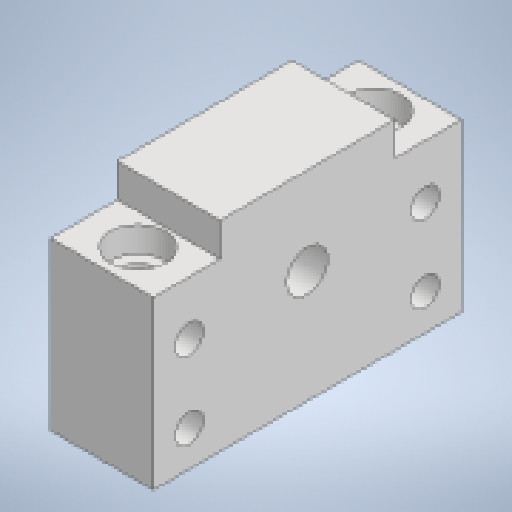
# Autodesk Inventor part: BF10
Saved by Autodesk Inventor 2023 (Build 270158000, 158)
## iProperties
Created: 2022-04-29
Part Number: BF10
Material: Generic
Document SubType Name: Modeling
Designer: plebbb
Density: 1 g/cm^3
Appearance: Default
Author: plebbb
Autodesk Inventor part; units mm, degrees
ref_plane "YZ Plane" through (0, 0, 0) normal (1, 0, 0) x (0, 1, 0)
ref_plane "XZ Plane" through (0, 0, 0) normal (0, 1, 0) x (-1, 0, 0)
ref_plane "XY Plane" through (0, 0, 0) normal (0, 0, 1) x (1, 0, 0)
sketch "Sketch1" plane through (0, 0, 0) normal (1, 0, 0) x (0, 1, 0)
  line L0 (0, 0) -> (32.5, 0)
  line L1 (32.5, 0) -> (32.5, -13)
  line L2 (32.5, -13) -> (39, -13)
  line L3 (39, -13) -> (39, -47)
  line L4 (39, -47) -> (32.5, -47)
  line L5 (32.5, -47) -> (32.5, -60)
  line L6 (32.5, -60) -> (0, -60)
  line L7 (0, -60) -> (0, 0)
  circle A0 centre (22, -53) radius 2.75
  circle A1 centre (7, -7) radius 2.75
  circle A2 centre (7, -53) radius 2.75
  circle A3 centre (22, -7) radius 2.75
  line L8 (22, -7) -> (7, -7) construction
  line L9 (7, -7) -> (7, -53) construction
  line L10 (7, -53) -> (22, -53) construction
  line L11 (22, -53) -> (22, -7) construction
  line L12 (7, -30) -> (0, -30) construction
  circle A4 centre (22, -30) radius 4
  dimension "d0" = 34
  dimension "d1" = 60
  dimension "d2" = 39
  dimension "d3" = 32.5
  dimension "d4" = 5.5
  dimension "d6" = 22
  dimension "d7" = 15
  dimension "d8" = 46
  dimension "d9" = 8
  constraints: 26 end point, 8 perpendicular, 5 centre point, 4 coincident, 4 midpoint, 3 equal radius, 2 horizontal, 2 parallel, 2 point on line, 1 collinear
  measures "d0" distance of L2.end L3.end
  measures "d1" distance between parallel lines of L6 L0
  measures "d2" distance between parallel lines of L7 L3
  measures "d3" distance from line of L0.start L1
  measures "d4" diameter of A3
  measures "d6" horizontal distance of L6.end A0.centre
  measures "d7" distance of L9.end L10.end
  measures "d8" distance of L8.end L9.end
  measures "d9" diameter of A4
extrude "Extrusion1" add sketch "Sketch1" along normal blind 20
sketch "Sketch2" plane through (0, 32.5, 0) normal (0, 1, 0) x (1, 0, 0)
  circle A0 centre (10, 7) radius 5.4
  circle A1 centre (10, 53) radius 5.4
  point P0 (0, 0)
  dimension "d12" = 10.8
  dimension "d13" = 10.8
  dimension "d14" = 46
  dimension "d15" = 7
  dimension "d16" = 10
  constraints: 2 centre point, 1 vertical alignment
  measures "d12" diameter of A0
  measures "d13" diameter of A1
  measures "d14" distance of A0.centre A1.centre
  measures "d15" vertical distance of point (0, 0) A0.centre
  measures "d16" horizontal distance of point (0, 0) A0.centre
extrude "Extrusion2" cut sketch "Sketch2" against normal blind 5
sketch "Sketch3" plane through (10, 27.5, -7) normal (0, 1, 0) x (1, 0, 0)
  circle A0 centre (0, 0) radius 5.4 projected
  circle A1 centre (0, 46) radius 5.4 projected
  circle A2 centre (0, 46) radius 3.3
  circle A3 centre (0, 0) radius 3.3
  point P0 (-10, -7)
  dimension "d19" = 6.6
  constraints: 2 centre point, 2 concentric, 1 equal radius
  measures "d19" diameter of A3
extrude "Extrusion3" cut sketch "Sketch3" against normal up to surface (27.5 mm away) contours A2 | A3
sketch "Sketch4" plane through (0, 0, 0) normal (-1, 0, 0) x (0, 0, 1)
  circle A0 centre (-30, 22) radius 11
  circle A1 centre (-30, 22) radius 4 projected
  point P0 (0, 0)
  dimension "d22" = 22
  constraints: 1 centre point, 1 concentric
  measures "d22" diameter of A0
extrude "Extrusion4" cut sketch "Sketch4" against normal blind 10
body "Solid1"
